Autodesk Fusion 360 part; units mm, degrees
(part 2 of 2)
sketch "Skizze4" plane through (0, 0, 5) normal (0, 0, 1) x (-1, 0, 0)
  arc A0 (299, -99.5) -> (300, -98.5) centre (299, -98.5) ccw
  line L0 (300, 67.5) -> (300, 98.5)
  arc A1 (300, 98.5) -> (299, 99.5) centre (299, 98.5) ccw
  line L1 (299, 99.5) -> (260.5, 99.5)
  arc A2 (259.5, 100.5) -> (260.5, 99.5) centre (260.5, 100.5) ccw
  line L2 (259.5, 100.5) -> (259.5, 139)
  arc A3 (259.5, 139) -> (258.5, 140) centre (258.5, 139) ccw
  line L3 (258.5, 140) -> (-258.5, 140)
  arc A4 (-258.5, 140) -> (-259.5, 139) centre (-258.5, 139) ccw
  line L4 (-259.5, 139) -> (-259.5, 100.5)
  arc A5 (-260.5, 99.5) -> (-259.5, 100.5) centre (-260.5, 100.5) ccw
  line L5 (-260.5, 99.5) -> (-299, 99.5)
  arc A6 (-299, 99.5) -> (-300, 98.5) centre (-299, 98.5) ccw
  line L6 (-300, 98.5) -> (-300, -98.5)
  arc A7 (-300, -98.5) -> (-299, -99.5) centre (-299, -98.5) ccw
  line L7 (-299, -99.5) -> (-260.5, -99.5)
  arc A8 (-259.5, -100.5) -> (-260.5, -99.5) centre (-260.5, -100.5) ccw
  line L8 (-259.5, -100.5) -> (-259.5, -139)
  arc A9 (-259.5, -139) -> (-258.5, -140) centre (-258.5, -139) ccw
  line L9 (-258.5, -140) -> (258.5, -140)
  arc A10 (258.5, -140) -> (259.5, -139) centre (258.5, -139) ccw
  line L10 (259.5, -139) -> (259.5, -100.5)
  arc A11 (260.5, -99.5) -> (259.5, -100.5) centre (260.5, -100.5) ccw
  line L11 (260.5, -99.5) -> (299, -99.5)
  circle A12 centre (65, 65) radius 4.25
  circle A13 centre (65, -65) radius 4.25
  circle A14 centre (-65, -65) radius 4.25
  circle A15 centre (-65, 65) radius 4.25
  line L12 (272.5, 67.5) -> (300, 67.5)
  line L13 (300, -98.5) -> (300, 12.5)
  line L14 (300, 12.5) -> (272.5, 12.5)
  arc A16 (272.5, 67.5) -> (272.5, 12.5) centre (272.5, 40) ccw

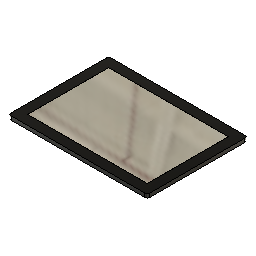
design "Tablet_Lenovo_X1"
Autodesk Fusion 360 part; units mm, degrees
sketch "Skizze1" plane through (0, 0, 0) normal (0, 0, 1) x (1, 0, 0)
  line L0 (-145.5, 105) -> (145.5, 105)
  line L1 (145.5, 105) -> (145.5, -105)
  line L2 (145.5, -105) -> (-145.5, -105)
  line L3 (-145.5, -105) -> (-145.5, 105)
  line L4 (-145.5, 105) -> (145.5, -105) construction
  line L5 (145.5, 105) -> (-145.5, -105) construction
  dimension "d1" = 291
  dimension "d2" = 210
  constraint horizontal L0
  constraint perpendicular L0 L1
  constraint parallel L0 L2
  constraint parallel L1 L3
  constraint coincident L4 origin
  constraint coincident L5 origin
  measures "d1" distance of L1.end L2.end
  measures "d2" distance of L0.end L1.end
extrude "Extrusion1" add sketch "Skizze1" along normal blind 8.9
chamfer "Fase1" distance 1 distance2 8.9 1 faces at (-48.5, -35, 0)
fillet "Abrundung1" radius 5 4 edges at (145, -104.5, 4.45) (145, 104.5, 4.45) (-145, -104.5, 4.45) (-145, 104.5, 4.45)
sketch "Skizze2" plane through (0, 0, 8.9) normal (0, 0, 1) x (-1, 0, 0)
  ellipse E0 centre (140.4685, -99.9685) end of major axis (144.0484, -103.5484) minor radius 5 (140.5313, -105) -> (145.5, -100.0313) ccw
  line L0 (145.5, -100.0313) -> (145.5, 100.0313)
  ellipse E1 centre (140.4685, 99.9685) end of major axis (144.0484, 103.5484) minor radius 5 (145.5, 100.0313) -> (140.5313, 105) ccw
  line L1 (140.5313, 105) -> (-140.5313, 105)
  ellipse E2 centre (-140.4685, 99.9685) end of major axis (-144.0484, 103.5484) minor radius 5 (-140.5313, 105) -> (-145.5, 100.0313) ccw
  line L2 (-145.5, 100.0313) -> (-145.5, -100.0313)
  ellipse E3 centre (-140.4685, -99.9685) end of major axis (-144.0484, -103.5484) minor radius 5 (-145.5, -100.0313) -> (-140.5313, -105) ccw
  line L3 (-140.5313, -105) -> (140.5313, -105)
  line L4 (125.5, -85) -> (-125.5, -85)
  line L5 (-125.5, -85) -> (-125.5, 85)
  line L6 (-125.5, 85) -> (125.5, 85)
  line L7 (125.5, 85) -> (125.5, -85)
  line L8 (125.5, -85) -> (-125.5, 85) construction
  line L9 (-125.5, -85) -> (125.5, 85) construction
  dimension "d9" = 20
  dimension "d10" = 20
  constraint horizontal L4
  constraint perpendicular L4 L5
  constraint parallel L4 L6
  constraint parallel L5 L7
  constraint coincident L8 origin
  constraint coincident L9 origin
  measures "d9" distance of L0 L7
  measures "d10" distance of L3 L4
extrude "Extrusion2" cut sketch "Skizze2" against normal blind 0.1 contours L4 L5 L6 L7
